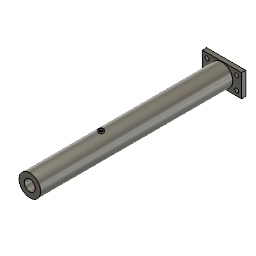
Full+System+Assembly (Autodesk Fusion 360 archive; units mm, degrees)
design "Measurement Tube"
Autodesk Fusion 360 part; units mm, degrees
note: some values were not read from the file. Set by a fixed rule: which face or edge a step refers to.
(part 1 of 5)
sketch "Sketch1" plane through (0, 0, 0) normal (0, 0, 1) x (1, 0, 0)
  circle A0 centre (0, 0) radius 6.375
  circle A1 centre (0, 0) radius 12.5
  dimension "d1" = 25
  dimension "d2" = 12.75
  constraint coincident A0.centre A1.centre
  measures "d1" diameter of A1
  measures "d2" diameter of A0
extrude "Extrude1" add sketch "Sketch1" along normal blind 225 contours A0 | A1
extrude "Extrude19" cut sketch "Sketch1" along normal up to surface (225 mm away) contours A0
sketch "Sketch22" plane through (0, 0, 0) normal (0, 0, 1) x (1, 0, 0)
  line L0 (22.5, 13) -> (-22.5, 13)
  line L1 (-22.5, 13) -> (-22.5, -13)
  line L2 (-22.5, -13) -> (22.5, -13)
  line L3 (22.5, -13) -> (22.5, 13)
  circle A0 centre (0, 0) radius 6.375 construction
  circle A1 centre (0, 0) radius 12.5 construction
  line L4 (0, 0) -> (22.5, 0) construction
  line L5 (0, 0) -> (-22.5, 0) construction
  circle A2 centre (0, 0) radius 12.5
  circle A3 centre (17, 7.5) radius 2.25
  circle A4 centre (-17, 7.5) radius 2.25
  circle A5 centre (-17, -7.5) radius 2.25
  circle A6 centre (17, -7.5) radius 2.25
  point P0 (12.5, 0)
  point P1 (-12.5, 0)
  dimension "d150" = 10
  dimension "d151" = 10
  dimension "d152" = 13
  dimension "d155" = 4.5
  dimension "d156" = 17
  dimension "d157" = 17
  dimension "d158" = 17
  dimension "d159" = 17
  dimension "d160" = 4.5
  dimension "d161" = 4.5
  dimension "d162" = 4.5
  dimension "d163" = 7.5
  dimension "d164" = 7.5
  dimension "d165" = 7.5
  dimension "d166" = 7.5
  constraint horizontal L0
  constraint vertical L1
  constraint horizontal L2
  constraint vertical L3
  constraint coincident A0.centre A1.centre
  constraint midpoint L3 L4.end
  constraint horizontal L4
  constraint coincident A1 P0
  constraint coincident L4 P0
  constraint midpoint L1 L5.end
  constraint coincident A1 P1
  constraint coincident L5 P1
  constraint coincident P0 A2
  measures "d150" distance of L4.end P0
  measures "d151" distance of L5.end P1
  measures "d152" distance of L0 A0.centre
  measures "d155" diameter of A3
  measures "d156" horizontal distance of A0.centre A3.centre
  measures "d157" horizontal distance of A0.centre A4.centre
  measures "d158" horizontal distance of A0.centre A6.centre
  measures "d159" horizontal distance of A0.centre A5.centre
  measures "d160" diameter of A4
  measures "d161" diameter of A6
  measures "d162" diameter of A5
  measures "d163" distance of L4 A3.centre
  measures "d164" distance of L5 A4.centre
  measures "d165" distance of L4 A6.centre
  measures "d166" distance of L5 A5.centre
extrude "Mount Holes" add sketch "Sketch22" along normal blind 5
ref_plane "WorkPlane4" through (0, 6.4, 0) normal (0, 1, 0) x (0, 0, 1)
sketch "Sketch21" plane through (0, 6.4, 0) normal (0, 1, 0) x (1, 0, 0)
  circle A0 centre (0, -143.363) radius 1.7
  circle A1 centre (0, -143.363) radius 2.7
  line L0 (-12.5, -225) -> (12.5, -225)
  line L1 (22.5, 0) -> (-22.5, 0) construction
  line L2 (-22.5, 0) -> (-22.5, -5) construction
  line L3 (-22.5, -5) -> (22.5, -5) construction
  line L4 (22.5, -5) -> (22.5, 0) construction
  line L5 (0, -5) -> (0, -225) construction
  dimension "d137" = 3.4
  dimension "d138" = 5.4
  dimension "d167" = 81.637
  constraint concentric A0 A1
  constraint midpoint L3 L5.start
  constraint midpoint L0 L5.end
  constraint coincident A0.centre L5
  measures "d137" diameter of A0
  measures "d138" diameter of A1
  measures "d167" distance of A0.centre L0
extrude "Extrude17" add sketch "Sketch21" along normal blind 8
extrude "Extrude18" cut sketch "Sketch21" along normal blind 8 and the other way blind 2 contours A0
equation "d5 = 12.8 mm"
equation "d20 = 0.105 in"
equation "d22 = d20"
equation "d29 = 2.5 in"
equation "d129 = 7.5 mm"
equation "d136 = d5 / 2"
equation "d138 = d137 + 2 mm"
equation "d151 = d150"
equation "d157 = d156"
equation "d158 = d156"
equation "d159 = d156"
equation "d160 = d155"
equation "d161 = d155"
equation "d162 = d155"
equation "d164 = d163"
equation "d165 = d163"
equation "d166 = d163"
equation "d50 = d48 / 2"
equation "d51 = d50"
equation "d52 = d53"
equation "d53 = d46 / 2"
equation "d54 = 4.25 mm"
equation "d55 = d54"
equation "d56 = -d45"
equation "d58 = 4.5 mm"
equation "d59 = d58"
equation "d64 = d67"
equation "d67 = 154.736 mm"
equation "d70 = d67"
equation "d110 = d26 / 2"
equation "d111 = d16 / 2"
equation "d115 = -d29"
equation "d119 = -d29"
equation "d127 = 17 mm"
equation "d128 = d127"
equation "d130 = d129"
equation "d131 = 4.25 mm"
equation "d132 = d131"

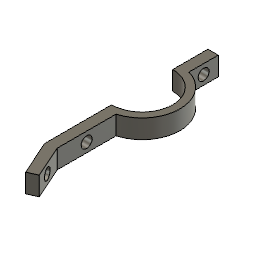
design "Trumpet Clamp 3 Secondary"
Autodesk Fusion 360 part; units mm, degrees
sketch "Sketch1" plane through (0, 0, 0) normal (0, 1, 0) x (1, 0, 0)
  circle A0 centre (0, 0) radius 12.435
  circle A1 centre (0, 0) radius 15.435
  line L0 (0, 0) -> (-15.435, 0) construction
  line L1 (0, 0) -> (15.435, 0) construction
  line L2 (-4.25, -40.647) -> (8.6182, -69.5153)
  line L3 (4.25, -38.8384) -> (16.3818, -66.0547)
  circle A2 centre (12.5, -67.785) radius 4.25
  line L4 (12.5, -67.785) -> (8.6182, -69.5153) construction
  line L5 (12.5, -67.785) -> (16.3818, -66.0547) construction
  circle A3 centre (12.5, -67.785) radius 2.25
  line L6 (-4.25, -40.647) -> (-4.25, -14.8384)
  line L7 (4.25, -38.8384) -> (4.25, -14.8384)
  line L8 (0, 0) -> (0, -38.8384) construction
  line L9 (4.25, -38.8384) -> (-4.25, -38.8384) construction
  line L10 (-4.25, 14.8384) -> (-4.25, 26.8384)
  line L11 (-4.25, 26.8384) -> (4.25, 26.8384)
  line L12 (4.25, 26.8384) -> (4.25, 14.8384)
  line L13 (-4.25, -14.8384) -> (-4.25, 14.8384) construction
  line L14 (4.25, 14.8384) -> (4.25, -14.8384) construction
  line L15 (12.5, -67.785) -> (12.5, -72.035) construction
  point P0 (0, -15.435)
  point P1 (12.5, -72.035)
  dimension "d1" = 24.87
  dimension "d3" = 4.5
  dimension "d4" = 8.5
  dimension "d5" = 12.5
  dimension "d19" = 8.5
  dimension "d22" = 30.87
  dimension "d31" = 12
  dimension "d32" = 24
  dimension "d35" = 56.6
  constraint coincident A0.centre A1.centre
  constraint concentric A0 A1
  constraint coincident A1 L0.end
  constraint horizontal L0
  constraint coincident A1 L1.end
  constraint parallel L0 L1
  constraint coincident A2.centre L4.start
  constraint coincident A2 L2.end
  constraint coincident A2 L3.end
  constraint parallel L4 L5
  constraint coincident L2.end L4.end
  constraint coincident L3.end L5.end
  constraint coincident A1 L6.end
  constraint coincident A1 L7.end
  constraint parallel L2 L3
  constraint vertical L6
  constraint vertical L7
  constraint vertical L8
  constraint tangent L3 A2
  constraint coincident L6 L9.end
  constraint perpendicular L6 L9
  constraint midpoint L8.end L9
  constraint coincident A1 L10.start
  constraint vertical L10
  constraint perpendicular L10 L11
  constraint coincident A1 L12.end
  constraint perpendicular L11 L12
  constraint vertical L13
  constraint vertical L14
  constraint coincident L8 P0
  constraint coincident A1 P0
  constraint coincident A2 P1
  constraint vertical L15
  constraint coincident P1 L15.end
  measures "d1" diameter of A0
  measures "d3" diameter of A3
  measures "d4" diameter of A2
  measures "d5" horizontal distance of A0.centre A2.centre
  measures "d19" distance of L6 L7
  measures "d22" diameter of A1
  measures "d31" distance of L11.end L12.end
  measures "d32" distance of L3.start L7.end
  measures "d35" vertical distance of P0 P1
extrude "Extrude1" add sketch "Sketch1" along normal blind 7.7
sketch "Sketch2" plane through (-10.8972, 0, 4.8575) normal (0.913367, 0, -0.407138) x (-0.407138, 0, -0.913367)
  line L0 (-67.0018, 0) -> (-37.204, 0)
  line L1 (-37.204, 0) -> (-37.204, 7.7)
  line L2 (-37.204, 7.7) -> (-67.0018, 7.7)
  line L3 (-67.0018, 7.7) -> (-67.0018, 0)
  line L4 (-37.204, 3.85) -> (-67.0018, 3.85) construction
  circle A0 centre (-45.204, 3.85) radius 2.25
  dimension "d33" = 8
  dimension "d34" = 4.5
  constraint midpoint L1 L4.start
  constraint midpoint L3 L4.end
  constraint coincident L4 A0.centre
  measures "d33" distance of L1 A0.centre
  measures "d34" diameter of A0
extrude "Extrude2" cut sketch "Sketch2" against normal up to surface (8.5 mm away) contours A0
sketch "Sketch3" plane through (4.25, 0, 0) normal (1, 0, 0) x (0, 0, -1)
  line L0 (-38.8384, 0) -> (-14.8384, 0)
  line L1 (-14.8384, 0) -> (-14.8384, 7.7)
  line L2 (-14.8384, 7.7) -> (-38.8384, 7.7)
  line L3 (-38.8384, 7.7) -> (-38.8384, 0)
  line L4 (-14.8384, 3.85) -> (-38.8384, 3.85) construction
  circle A0 centre (-26.8384, 3.85) radius 2.25
  line L5 (14.8384, 0) -> (26.8384, 0) construction
  line L6 (26.8384, 0) -> (26.8384, 7.7) construction
  line L7 (26.8384, 7.7) -> (14.8384, 7.7) construction
  line L8 (14.8384, 7.7) -> (14.8384, 0) construction
  line L9 (14.8384, 3.85) -> (26.8384, 3.85) construction
  circle A1 centre (20.8384, 3.85) radius 2.25
  dimension "d16" = 4.5
  constraint midpoint L1 L4.start
  constraint midpoint L3 L4.end
  constraint midpoint L4 A0.centre
  constraint midpoint L8 L9.start
  constraint midpoint L6 L9.end
  constraint midpoint L9 A1.centre
  constraint equal A0 A1
  measures "d16" diameter of A0
extrude "Extrude3" cut sketch "Sketch3" against normal up to surface (8.5 mm away) contours A0 | A1
sketch "Sketch4" plane through (0, 0, 0) normal (1, 0, 0) x (0, 0, -1)
  circle A0 centre (-26.8384, 3.85) radius 2.25 construction
  line L0 (-38.8384, 0) -> (-14.8384, 0) construction
  line L1 (-14.8384, 0) -> (-14.8384, 7.7) construction
  line L2 (-14.8384, 7.7) -> (-38.8384, 7.7) construction
  line L3 (-38.8384, 7.7) -> (-38.8384, 0) construction
  line L4 (14.8384, 0) -> (-14.8384, 0) construction
  line L5 (-14.8384, 0) -> (-14.8384, 7.7) construction
  line L6 (14.8384, 7.7) -> (-14.8384, 7.7) construction
  line L7 (-14.8384, 7.7) -> (-14.8384, 0) construction
  circle A1 centre (-26.8384, 3.85) radius 2.25 construction
  line L8 (-14.8384, 0) -> (-40.647, 0) construction
  line L9 (-40.647, 0) -> (-40.647, 7.7) construction
  line L10 (-40.647, 7.7) -> (-14.8384, 7.7) construction
  line L11 (-14.8384, 7.7) -> (-14.8384, 0) construction
  line L12 (14.8384, 0) -> (-39.7427, 0)
  line L13 (-39.7427, 0) -> (-39.7427, 7.7)
  line L14 (-39.7427, 7.7) -> (14.8384, 7.7)
  line L15 (14.8384, 7.7) -> (14.8384, 0)
  line L16 (-40.647, 7.7) -> (-38.8384, 7.7) construction
  line L17 (14.8384, 7.7) -> (14.8384, 0)
  line L18 (14.8384, 0) -> (-14.8384, 0)
  line L19 (14.8384, 0) -> (14.8384, 7.7)
  line L20 (14.8384, 7.7) -> (-14.8384, 7.7)
  circle A2 centre (20.8384, 3.85) radius 2.25
  line L21 (14.8384, 0) -> (26.8384, 0)
  line L22 (26.8384, 0) -> (26.8384, 7.7)
  line L23 (26.8384, 7.7) -> (14.8384, 7.7)
  line L24 (14.8384, 7.7) -> (14.8384, 0)
  constraint horizontal L12
  constraint vertical L13
  constraint horizontal L14
  constraint vertical L15
  constraint coincident L10 L13.end
  constraint coincident L4.start L12.start
  constraint coincident L9.end L10.start
  constraint coincident L2.end L3.start
  constraint midpoint L13.end L16
extrude "Extrude4" cut sketch "Sketch4" against normal blind 15.435
ref_plane "WorkPlane1" through (6.0659, 3.85, 53.3509) normal (-0.913367, 0, 0.407138) x (0.407138, 0, 0.913367)
sketch "Sketch5" plane through (-14.779, 0, 6.5878) normal (-0.913367, 0, 0.407138) x (0.407138, 0, 0.913367)
  line L0 (11.3577, 7.7) -> (11.3577, 0) construction
  line L1 (11.3577, 0) -> (36.2997, 0) construction
  line L2 (36.2997, 0) -> (36.2997, 7.7) construction
  line L3 (36.2997, 7.7) -> (11.3577, 7.7) construction
  ellipse E0 centre (24.5133, 3.85) end of major axis (24.5133, 1.6) minor radius 2.0551
  line L4 (64.7518, 7.7) -> (69.2518, 7.7) construction
  line L5 (36.2997, 7.7) -> (67.0018, 7.7) construction
  line L6 (67.0018, 7.7) -> (67.0018, 0) construction
  line L7 (67.0018, 0) -> (36.2997, 0) construction
  line L8 (36.2997, 0) -> (36.2997, 7.7) construction
  line L9 (51.6507, 7.7) -> (33.5308, 7.7)
  line L10 (33.5308, 7.7) -> (33.5308, 0)
  line L11 (33.5308, 0) -> (51.6507, 0)
  line L12 (51.6507, 0) -> (51.6507, 7.7)
  constraint horizontal L5
  constraint vertical L6
  constraint horizontal L7
  constraint vertical L8
  constraint coincident L2.end L3.start
  constraint midpoint L4 L5.end
  constraint coincident L1.end L7
  constraint horizontal L9
  constraint vertical L10
  constraint horizontal L11
  constraint vertical L12
  constraint coincident L1 L10.end
  constraint midpoint L5 L9.start
extrude "Extrude5" cut sketch "Sketch5" along normal up to surface (4.25 mm away) contours L9 L10 L11 L12
sketch "Sketch6" plane through (-18.6608, 0, 8.3181) normal (-0.913367, 0, 0.407138) x (0.407138, 0, 0.913367)
  line L0 (36.2997, 7.7) -> (36.2997, 0)
  line L1 (36.2997, 0) -> (51.6507, 0)
  line L2 (51.6507, 7.7) -> (36.2997, 7.7)
  circle A0 centre (45.204, 3.85) radius 2.25
  line L3 (51.6507, 7.7) -> (111.7151, 7.7)
  line L4 (111.7151, 7.7) -> (111.7151, 0)
  line L5 (111.7151, 0) -> (51.6507, 0)
  line L6 (51.6507, 0) -> (51.6507, 7.7)
  line L7 (51.6507, 0) -> (51.6507, 7.7)
  constraint horizontal L3
  constraint vertical L4
  constraint horizontal L5
  constraint vertical L6
  constraint coincident L2.start L3.start
  constraint coincident L1.end L5
extrude "Extrude6" cut sketch "Sketch6" against normal up to surface (8.5 mm away) contours L3 L4 L5 L6 L7
equation "d19 = d4"
equation "d20 = ( -d22 / 2 mm ) * 1 mm"
equation "d22 = d1 + 6 mm"

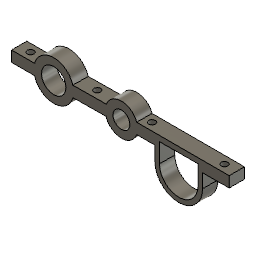
design "Trumpet Mount Close"
Autodesk Fusion 360 part; units mm, degrees
sketch "Sketch1" plane through (0, 0, 0) normal (0, 0, 1) x (1, 0, 0)
  circle A0 centre (-43.925, 0) radius 12.925
  circle A1 centre (-43.925, 0) radius 7.925
  circle A2 centre (0, 0) radius 10.5
  circle A3 centre (0, 0) radius 5.5
  line L0 (9.8995, 3.5) -> (69.8995, 3.5)
  line L1 (69.8995, 3.5) -> (69.8995, -3.5)
  line L2 (69.8995, -3.5) -> (9.8995, -3.5)
  line L3 (-31.5162, 3.6163) -> (-9.7806, 3.8197)
  line L4 (-31.4507, -3.3834) -> (-10.006, -3.1827)
  line L5 (-56.3671, 3.5) -> (-71.3671, 3.5)
  line L6 (-71.3671, 3.5) -> (-71.3671, -3.5)
  line L7 (-71.3671, -3.5) -> (-56.3671, -3.5)
  line L8 (-43.925, 0) -> (0, 0) construction
  dimension "d1" = 3.5
  dimension "d2" = 3.5
  dimension "d3" = 3.5
  dimension "d4" = 3.5
  dimension "d5" = 3.5
  dimension "d6" = 3.5
  dimension "d7" = 43.925
  dimension "d8" = 60
  dimension "d9" = 15
  dimension "d19" = 25.85
  dimension "d20" = 21
  dimension "d21" = 11
  dimension "d22" = 15.85
  constraint concentric A0 A1
  constraint concentric A2 A3
  constraint coincident A2 L0.start
  constraint horizontal L0
  constraint perpendicular L0 L1
  constraint coincident A2 L2.end
  constraint perpendicular L1 L2
  constraint coincident A0 L3.start
  constraint coincident A2 L3.end
  constraint coincident A0 L4.start
  constraint coincident A2 L4.end
  constraint parallel L3 L4
  constraint coincident A0 L5.start
  constraint horizontal L5
  constraint perpendicular L5 L6
  constraint coincident A0 L7.end
  constraint perpendicular L6 L7
  constraint coincident A0.centre A1.centre
  constraint coincident A2.centre A3.centre
  constraint horizontal L8
  measures "d1" distance of A2.centre L2
  measures "d2" distance of A2.centre L0
  measures "d3" distance of A0.centre L3
  measures "d4" distance of A0.centre L4
  measures "d5" distance of A0.centre L7
  measures "d6" distance of A0.centre L5
  measures "d7" horizontal distance of A0.centre A2.centre
  measures "d8" distance of L0.start L0.end
  measures "d9" distance of L5.start L5.end
  measures "d19" diameter of A0
  measures "d20" diameter of A2
  measures "d21" diameter of A3
  measures "d22" diameter of A1
extrude "Extrude1" add sketch "Sketch1" along normal mid plane 10
sketch "Sketch4" plane through (0, 3.5, 0) normal (0, 1, 0) x (-1, 0, 0)
  line L0 (71.3671, -5) -> (71.3671, 5)
  line L1 (71.3671, 5) -> (56.3671, 5)
  line L2 (56.3671, 5) -> (56.3671, -5)
  line L3 (56.3671, -5) -> (71.3671, -5)
  circle A0 centre (63.8671, 0) radius 2.125
  line L4 (31.5162, -5) -> (9.7806, -5)
  line L5 (31.5162, 5) -> (31.5162, -5)
  line L6 (9.7806, -5) -> (9.7806, 5)
  dimension "d25" = 4.25
  dimension "d27" = 5
  dimension "d31" = 7.5
  dimension "d32" = 7.5
  measures "d25" diameter of A0
  measures "d27" distance of L3 A0.centre
  measures "d31" distance of L0 A0.centre
  measures "d32" distance of L2 A0.centre
extrude "Extrude4" cut sketch "Sketch4" along normal up to surface contours A0 end surface through (-31.4507, -3.3834, 0) normal (0.009359, -0.999956, 0) offset 0
sketch "Sketch5" plane through (-0.0366, 3.9109, 0) normal (-0.009359, 0.999956, 0) x (0, 0, 1)
  line L0 (-5, -31.481) -> (5, -31.481)
  line L1 (5, -31.481) -> (5, -9.7444)
  line L2 (5, -9.7444) -> (-5, -9.7444)
  line L3 (-5, -9.7444) -> (-5, -31.481)
  circle A0 centre (0, -20.613) radius 2.125
  dimension "d35" = 4.25
  dimension "d36" = 10.868
  dimension "d37" = 10.8686
  dimension "d38" = 5
  measures "d35" diameter of A0
  measures "d36" distance of L0 A0.centre
  measures "d37" distance of L2 A0.centre
  measures "d38" distance of L3 A0.centre
extrude "Extrude5" cut sketch "Sketch5" against normal up to surface (7 mm away) contours A0
sketch "Sketch6" plane through (0, 3.5, 0) normal (0, 1, 0) x (-1, 0, 0)
  line L0 (-9.8995, -5) -> (-9.8995, 5)
  line L1 (-9.8995, 5) -> (-69.8995, 5)
  line L2 (-69.8995, 5) -> (-69.8995, -5)
  line L3 (-69.8995, -5) -> (-9.8995, -5)
sketch "Sketch7" plane through (0, 3.5, 0) normal (0, 1, 0) x (-1, 0, 0)
  line L0 (-9.8995, -5) -> (-9.8995, 5) construction
  line L1 (-9.8995, 5) -> (-69.8995, 5) construction
  line L2 (-69.8995, 5) -> (-69.8995, -5) construction
  line L3 (-69.8995, -5) -> (-9.8995, -5) construction
  line L4 (-69.8995, 0) -> (-9.8995, 0) construction
  circle A0 centre (-61.8995, 0) radius 2.125
  circle A1 centre (-14.8995, 0) radius 2.125
  dimension "d41" = 4.25
  dimension "d42" = 4.25
  dimension "d43" = 8
  dimension "d44" = 5
  constraint midpoint L2 L4.start
  constraint midpoint L0 L4.end
  constraint coincident L4 A0.centre
  constraint coincident L4 A1.centre
  measures "d41" diameter of A0
  measures "d42" diameter of A1
  measures "d43" distance of L2 A0.centre
  measures "d44" distance of L0 A1.centre
extrude "Extrude6" cut sketch "Sketch7" against normal up to surface (7 mm away)
sketch "Sketch8" plane through (0, 0, 5) normal (0, 0, 1) x (1, 0, 0)
  line L0 (-71.3671, 3.5) -> (-71.3671, -3.5)
  line L1 (-71.3671, -3.5) -> (-56.3671, -3.5)
  arc A0 (-56.3671, -3.5) -> (-31.4507, -3.3834) centre (-43.925, 0) ccw
  line L2 (-31.4507, -3.3834) -> (-10.006, -3.1827)
  arc A1 (-10.006, -3.1827) -> (9.8995, -3.5) centre (0, 0) ccw
  line L3 (9.8995, -3.5) -> (69.8995, -3.5)
  line L4 (69.8995, -3.5) -> (69.8995, 3.5)
  line L5 (52.6495, 0) -> (52.6495, -28) construction
  line L6 (52.6495, -28) -> (21.6495, -28) construction
  line L7 (21.6495, -28) -> (21.6495, 0) construction
  circle A2 centre (37.1495, -12.5) radius 12.5 construction
  line L8 (37.1495, -12.5) -> (37.1495, 0) construction
  line L9 (37.1495, -12.5) -> (52.6495, -12.5) construction
  line L10 (37.1495, -12.5) -> (21.6495, -12.5) construction
  line L11 (24.6495, -12.5) -> (24.6495, 0)
  line L12 (49.6495, -12.5) -> (49.6495, 0)
  arc A3 (24.6495, -12.5) -> (49.6495, -12.5) centre (37.1495, -12.5) ccw
  arc A4 (21.6495, -12.5) -> (37.1495, -28) centre (37.1495, -12.5) ccw
  arc A5 (37.1495, -28) -> (52.6495, -12.5) centre (37.1495, -12.5) ccw
  line L13 (21.6495, -12.5) -> (21.6495, 0)
  line L14 (52.6495, -12.5) -> (52.6495, 0)
  line L15 (21.6495, 0) -> (52.6495, 0)
  circle A6 centre (-43.925, 0) radius 7.925
  circle A7 centre (0, 0) radius 5.5
  arc A8 (-31.5162, 3.6163) -> (-56.3671, 3.5) centre (-43.925, 0) ccw
  line L16 (-56.3671, 3.5) -> (-71.3671, 3.5)
  line L17 (69.8995, 3.5) -> (9.8995, 3.5)
  arc A9 (9.8995, 3.5) -> (-9.7806, 3.8197) centre (0, 0) ccw
  line L18 (-9.7806, 3.8197) -> (-31.5162, 3.6163)
  point P0 (37.1495, 0)
  dimension "d49" = 17.25
  dimension "d50" = 31
  dimension "d51" = 28
  dimension "d52" = 25
  constraint vertical L5
  constraint horizontal L6
  constraint vertical L7
  constraint coincident A2.centre L8.start
  constraint coincident L8 P0
  constraint coincident A2 P0
  constraint coincident L5 L9.end
  constraint perpendicular L5 L9
  constraint coincident L7 L10.end
  constraint perpendicular L7 L10
  constraint coincident A2 L11.start
  constraint coincident L10 L11.start
  constraint tangent A2 L11
  constraint coincident A2 L12.start
  constraint coincident L9 L12.start
  constraint tangent A2 L12
  constraint tangent L12 A3
  constraint tangent L6 A4
  constraint coincident L6 A4.end
  constraint tangent L5 A5
  constraint perpendicular L14 L15
  constraint coincident L11.end L15
  constraint coincident L12.end L15
  constraint coincident P0 L15
  constraint midpoint P0 L15
  measures "d49" distance of L4 L5
  measures "d50" distance of L7.end L5.start
  measures "d51" distance of L5.start L5.end
  measures "d52" diameter of A2
extrude "Extrude7" add sketch "Sketch8" against normal up to surface (10 mm away) contours L3 L11 L12 A3 A4 A5 L13 L14
sketch "Sketch9" plane through (0, 0, 5) normal (0, 0, 1) x (1, 0, 0)
  line L0 (24.6495, -3.5) -> (49.6495, -3.5)
  line L1 (49.6495, -3.5) -> (49.6495, -12.5)
  arc A0 (24.6495, -12.5) -> (49.6495, -12.5) centre (37.1495, -12.5) ccw
  line L2 (24.6495, -12.5) -> (24.6495, -3.5)
  line L3 (21.6495, -3.5) -> (21.6495, -12.5)
  arc A1 (21.6495, -12.5) -> (37.1495, -28) centre (37.1495, -12.5) ccw
  line L4 (52.6495, -12.5) -> (52.6495, -3.5)
  line L5 (52.6495, -3.5) -> (69.8995, -3.5)
  line L6 (69.8995, -3.5) -> (69.8995, 3.5)
  line L7 (-71.3671, 3.5) -> (-71.3671, -3.5)
  line L8 (-71.3671, -3.5) -> (-56.3671, -3.5)
  arc A2 (-56.3671, -3.5) -> (-31.4507, -3.3834) centre (-43.925, 0) ccw
  line L9 (-31.4507, -3.3834) -> (-10.006, -3.1827)
  arc A3 (-10.006, -3.1827) -> (9.8995, -3.5) centre (0, 0) ccw
  line L10 (9.8995, -3.5) -> (21.6495, -3.5)
  line L11 (24.6495, -3.5) -> (49.6495, -3.5)
  line L12 (49.6495, -3.5) -> (49.6495, 0)
  line L13 (49.6495, 0) -> (24.6495, 0)
  line L14 (24.6495, 0) -> (24.6495, -3.5)
  line L15 (49.6495, -6.9259) -> (49.6495, 0) construction
  arc A4 (37.1495, -28) -> (52.6495, -12.5) centre (37.1495, -12.5) ccw
  circle A5 centre (-43.925, 0) radius 7.925
  circle A6 centre (0, 0) radius 5.5
  line L16 (69.8995, 3.5) -> (9.8995, 3.5)
  arc A7 (9.8995, 3.5) -> (-9.7806, 3.8197) centre (0, 0) ccw
  line L17 (-9.7806, 3.8197) -> (-31.5162, 3.6163)
  arc A8 (-31.5162, 3.6163) -> (-56.3671, 3.5) centre (-43.925, 0) ccw
  line L18 (-56.3671, 3.5) -> (-71.3671, 3.5)
  constraint horizontal L11
  constraint vertical L12
  constraint horizontal L13
  constraint vertical L14
  constraint coincident L0.start L2.end
  constraint coincident L1 L15.start
  constraint perpendicular L13 L15
extrude "Extrude8" cut sketch "Sketch9" against normal up to surface (10 mm away) contours L0 L11 L12 L13 L14
sketch "Sketch3" plane through (0, 0, 0) normal (0, 1, 0) x (1, 0, 0)
  line L0 (-71.3671, 5) -> (-71.3671, -5)
  line L1 (-71.3671, -5) -> (-56.3671, -5)
  line L2 (-56.3671, -5) -> (-56.3671, 5)
  line L3 (-56.3671, 5) -> (-71.3671, 5)
  line L4 (9.8995, 5) -> (9.8995, -5)
  line L5 (9.8995, -5) -> (69.8995, -5)
  line L6 (69.8995, -5) -> (69.8995, 5)
  line L7 (69.8995, 5) -> (9.8995, 5)
  line L8 (-71.3671, 5) -> (69.8995, 5)
  line L9 (69.8995, 5) -> (69.8995, -5)
  line L10 (69.8995, -5) -> (-71.3671, -5)
  line L11 (-71.3671, -5) -> (-71.3671, 5)
  circle A0 centre (-63.8671, 0) radius 2.125
  circle A1 centre (14.8995, 0) radius 2.125
  circle A2 centre (61.8995, 0) radius 2.125
  constraint horizontal L8
  constraint vertical L9
  constraint horizontal L10
  constraint vertical L11
  constraint coincident L5.end L6.start
  constraint coincident L0.start L3.end
extrude "Extrude3" [rolled back] along distance 20 taper angle 0
equation "d2 = d1"
equation "d3 = d1"
equation "d4 = d1"
equation "d5 = d1"
equation "d6 = d1"
equation "d42 = d41"
equation "d49 = 20.25 mm - 3 mm"
equation "d50 = 25 mm + 6 mm"
equation "d51 = 25 mm + 3 mm"

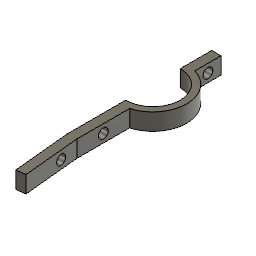
design "Trumpet Clamp 2 Secondary"
Autodesk Fusion 360 part; units mm, degrees
sketch "Sketch1" plane through (0, 0, 0) normal (0, 1, 0) x (1, 0, 0)
  circle A0 centre (0, 0) radius 12.435
  circle A1 centre (0, 0) radius 15.435
  line L0 (0, 0) -> (-15.435, 0) construction
  line L1 (0, 0) -> (15.435, 0) construction
  line L2 (-4.25, -39.2475) -> (0.7697, -91.2632)
  line L3 (4.25, -38.8384) -> (9.2303, -90.4468)
  circle A2 centre (5, -90.855) radius 4.25
  line L4 (5, -90.855) -> (0.7697, -91.2632) construction
  line L5 (5, -90.855) -> (9.2303, -90.4468) construction
  circle A3 centre (5, -90.855) radius 2.25
  line L6 (-4.25, -39.2475) -> (-4.25, -14.8384)
  line L7 (4.25, -38.8384) -> (4.25, -14.8384)
  line L8 (0, 0) -> (0, -38.8384) construction
  line L9 (4.25, -38.8384) -> (-4.25, -38.8384) construction
  line L10 (-4.25, 14.8384) -> (-4.25, 26.8384)
  line L11 (-4.25, 26.8384) -> (4.25, 26.8384)
  line L12 (4.25, 26.8384) -> (4.25, 14.8384)
  line L13 (-4.25, -14.8384) -> (-4.25, 14.8384) construction
  line L14 (4.25, 14.8384) -> (4.25, -14.8384) construction
  line L15 (5, -90.855) -> (5, -95.105) construction
  point P0 (0, -15.435)
  point P1 (5, -95.105)
  dimension "d1" = 24.87
  dimension "d3" = 4.5
  dimension "d4" = 8.5
  dimension "d5" = 5
  dimension "d19" = 8.5
  dimension "d22" = 30.87
  dimension "d31" = 12
  dimension "d32" = 24
  dimension "d35" = 79.67
  constraint coincident A0.centre A1.centre
  constraint concentric A0 A1
  constraint coincident A1 L0.end
  constraint horizontal L0
  constraint coincident A1 L1.end
  constraint parallel L0 L1
  constraint coincident A2.centre L4.start
  constraint coincident A2 L2.end
  constraint coincident A2 L3.end
  constraint parallel L4 L5
  constraint coincident L2.end L4.end
  constraint coincident L3.end L5.end
  constraint coincident A1 L6.end
  constraint coincident A1 L7.end
  constraint parallel L2 L3
  constraint vertical L6
  constraint vertical L7
  constraint vertical L8
  constraint tangent L3 A2
  constraint coincident L6 L9.end
  constraint perpendicular L6 L9
  constraint midpoint L8.end L9
  constraint coincident A1 L10.start
  constraint vertical L10
  constraint perpendicular L10 L11
  constraint coincident A1 L12.end
  constraint perpendicular L11 L12
  constraint vertical L13
  constraint vertical L14
  constraint coincident L8 P0
  constraint coincident A1 P0
  constraint coincident A2 P1
  constraint vertical L15
  constraint coincident P1 L15.end
  measures "d1" diameter of A0
  measures "d3" diameter of A3
  measures "d4" diameter of A2
  measures "d5" horizontal distance of A0.centre A2.centre
  measures "d19" distance of L6 L7
  measures "d22" diameter of A1
  measures "d31" distance of L11.end L12.end
  measures "d32" distance of L3.start L7.end
  measures "d35" vertical distance of P0 P1
extrude "Extrude1" add sketch "Sketch1" along normal blind 7.7
sketch "Sketch2" plane through (0.4974, 0, -0.048) normal (0.995376, 0, -0.096056) x (-0.096056, 0, -0.995376)
  line L0 (-90.9152, 0) -> (-39.067, 0)
  line L1 (-39.067, 0) -> (-39.067, 7.7)
  line L2 (-39.067, 7.7) -> (-90.9152, 7.7)
  line L3 (-90.9152, 7.7) -> (-90.9152, 0)
  line L4 (-39.067, 3.85) -> (-90.9152, 3.85) construction
  circle A0 centre (-47.067, 3.85) radius 2.25
  dimension "d33" = 8
  dimension "d34" = 4.5
  constraint midpoint L1 L4.start
  constraint midpoint L3 L4.end
  constraint coincident L4 A0.centre
  measures "d33" distance of L1 A0.centre
  measures "d34" diameter of A0
extrude "Extrude2" cut sketch "Sketch2" against normal up to surface (8.5 mm away) contours A0
sketch "Sketch3" plane through (4.25, 0, 0) normal (1, 0, 0) x (0, 0, -1)
  line L0 (-38.8384, 0) -> (-14.8384, 0)
  line L1 (-14.8384, 0) -> (-14.8384, 7.7)
  line L2 (-14.8384, 7.7) -> (-38.8384, 7.7)
  line L3 (-38.8384, 7.7) -> (-38.8384, 0)
  line L4 (-14.8384, 3.85) -> (-38.8384, 3.85) construction
  circle A0 centre (-26.8384, 3.85) radius 2.25
  line L5 (14.8384, 0) -> (26.8384, 0) construction
  line L6 (26.8384, 0) -> (26.8384, 7.7) construction
  line L7 (26.8384, 7.7) -> (14.8384, 7.7) construction
  line L8 (14.8384, 7.7) -> (14.8384, 0) construction
  line L9 (14.8384, 3.85) -> (26.8384, 3.85) construction
  circle A1 centre (20.8384, 3.85) radius 2.25
  dimension "d16" = 4.5
  constraint midpoint L1 L4.start
  constraint midpoint L3 L4.end
  constraint midpoint L4 A0.centre
  constraint midpoint L8 L9.start
  constraint midpoint L6 L9.end
  constraint midpoint L9 A1.centre
  constraint equal A0 A1
  measures "d16" diameter of A0
extrude "Extrude3" cut sketch "Sketch3" against normal up to surface (8.5 mm away) contours A0 | A1
sketch "Sketch4" plane through (0, 0, 0) normal (1, 0, 0) x (0, 0, -1)
  circle A0 centre (-26.8384, 3.85) radius 2.25 construction
  line L0 (-38.8384, 0) -> (-14.8384, 0) construction
  line L1 (-14.8384, 0) -> (-14.8384, 7.7) construction
  line L2 (-14.8384, 7.7) -> (-38.8384, 7.7) construction
  line L3 (-38.8384, 7.7) -> (-38.8384, 0) construction
  line L4 (14.8384, 0) -> (-14.8384, 0) construction
  line L5 (-14.8384, 0) -> (-14.8384, 7.7) construction
  line L6 (14.8384, 7.7) -> (-14.8384, 7.7) construction
  line L7 (-14.8384, 7.7) -> (-14.8384, 0) construction
  circle A1 centre (-26.8384, 3.85) radius 2.25 construction
  line L8 (-14.8384, 0) -> (-39.2475, 0) construction
  line L9 (-39.2475, 0) -> (-39.2475, 7.7) construction
  line L10 (-39.2475, 7.7) -> (-14.8384, 7.7) construction
  line L11 (-14.8384, 7.7) -> (-14.8384, 0) construction
  line L12 (14.8384, 0) -> (-39.0429, 0)
  line L13 (-39.0429, 0) -> (-39.0429, 7.7)
  line L14 (-39.0429, 7.7) -> (14.8384, 7.7)
  line L15 (14.8384, 7.7) -> (14.8384, 0)
  line L16 (-39.2475, 7.7) -> (-38.8384, 7.7) construction
  line L17 (14.8384, 7.7) -> (14.8384, 0)
  line L18 (14.8384, 0) -> (-14.8384, 0)
  line L19 (14.8384, 0) -> (14.8384, 7.7)
  line L20 (14.8384, 7.7) -> (-14.8384, 7.7)
  circle A2 centre (20.8384, 3.85) radius 2.25
  line L21 (14.8384, 0) -> (26.8384, 0)
  line L22 (26.8384, 0) -> (26.8384, 7.7)
  line L23 (26.8384, 7.7) -> (14.8384, 7.7)
  line L24 (14.8384, 7.7) -> (14.8384, 0)
  constraint horizontal L12
  constraint vertical L13
  constraint horizontal L14
  constraint vertical L15
  constraint coincident L10 L13.end
  constraint coincident L4.start L12.start
  constraint coincident L9.end L10.start
  constraint coincident L2.end L3.start
  constraint midpoint L13.end L16
extrude "Extrude4" cut sketch "Sketch4" against normal blind 15.435
ref_plane "WorkPlane1" through (2.4902, 3.85, 64.8471) normal (-0.995376, 0, 0.096056) x (0.096056, 0, 0.995376)
sketch "Sketch5" plane through (-3.733, 0, 0.3602) normal (-0.995376, 0, 0.096056) x (0.096056, 0, 0.995376)
  line L0 (12.3775, 7.7) -> (12.3775, 0) construction
  line L1 (12.3775, 0) -> (38.8624, 0) construction
  line L2 (38.8624, 0) -> (38.8624, 7.7) construction
  line L3 (38.8624, 7.7) -> (12.3775, 7.7) construction
  ellipse E0 centre (26.7142, 3.85) end of major axis (26.7142, 1.6) minor radius 2.2396
  line L4 (88.6652, 7.7) -> (93.1652, 7.7) construction
  line L5 (38.8624, 7.7) -> (90.9152, 7.7) construction
  line L6 (90.9152, 7.7) -> (90.9152, 0) construction
  line L7 (90.9152, 0) -> (38.8624, 0) construction
  line L8 (38.8624, 0) -> (38.8624, 7.7) construction
  line L9 (64.8888, 7.7) -> (33.5308, 7.7)
  line L10 (33.5308, 7.7) -> (33.5308, 0)
  line L11 (33.5308, 0) -> (64.8888, 0)
  line L12 (64.8888, 0) -> (64.8888, 7.7)
  constraint horizontal L5
  constraint vertical L6
  constraint horizontal L7
  constraint vertical L8
  constraint coincident L2.end L3.start
  constraint midpoint L4 L5.end
  constraint coincident L1.end L7
  constraint horizontal L9
  constraint vertical L10
  constraint horizontal L11
  constraint vertical L12
  constraint coincident L1 L10.end
  constraint midpoint L5 L9.start
extrude "Extrude5" cut sketch "Sketch5" along normal up to surface (4.25 mm away) contours L9 L10 L11 L12
sketch "Sketch6" plane through (-7.9633, 0, 0.7685) normal (-0.995376, 0, 0.096056) x (0.096056, 0, 0.995376)
  line L0 (38.8624, 7.7) -> (38.8624, 0)
  line L1 (38.8624, 0) -> (64.8888, 0)
  line L2 (64.8888, 7.7) -> (38.8624, 7.7)
  circle A0 centre (47.067, 3.85) radius 2.25
  line L3 (64.8888, 7.7) -> (111.7152, 7.7)
  line L4 (111.7152, 7.7) -> (111.7152, 0)
  line L5 (111.7152, 0) -> (64.8888, 0)
  line L6 (64.8888, 0) -> (64.8888, 7.7)
  line L7 (64.8888, 0) -> (64.8888, 7.7)
  constraint horizontal L3
  constraint vertical L4
  constraint horizontal L5
  constraint vertical L6
  constraint coincident L2.start L3.start
  constraint coincident L1.end L5
extrude "Extrude6" cut sketch "Sketch6" against normal up to surface (8.5 mm away) contours L3 L4 L5 L6 L7
equation "d19 = d4"
equation "d20 = ( -d22 / 2 mm ) * 1 mm"
equation "d22 = d1 + 6 mm"

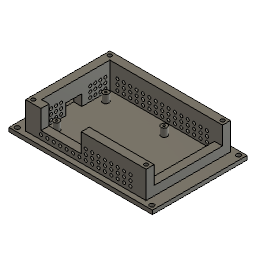
design "RPi Board Case"
Autodesk Fusion 360 part; units mm, degrees
sketch "Sketch1" plane through (0, 0, 0) normal (0, 1, 0) x (1, 0, 0)
  line L0 (-60, 42) -> (60, 42)
  line L1 (60, 42) -> (60, -42)
  line L2 (60, -42) -> (-60, -42)
  line L3 (-60, -42) -> (-60, 42)
  dimension "d1" = 120
  dimension "d2" = 84
  dimension "d3" = 60
  dimension "d4" = 42
  constraint horizontal L0
  constraint vertical L1
  constraint horizontal L2
  constraint vertical L3
  measures "d1" distance of L0.start L0.end
  measures "d2" distance of L0.start L2.end
  measures "d3" distance of origin L1
  measures "d4" distance of origin L0
extrude "Extrude1" add sketch "Sketch1" along normal blind 5 makes body 1
sketch "Sketch2" plane through (0, 5, 0) normal (0, 1, 0) x (-1, 0, 0)
  line L0 (60, 42) -> (-60, 42)
  line L1 (-60, 42) -> (-60, -42)
  line L2 (-60, -42) -> (60, -42)
  line L3 (60, -42) -> (60, 42)
  line L4 (52, -34) -> (-52, -34)
  line L5 (-52, -34) -> (-52, 34)
  line L6 (-52, 34) -> (52, 34)
  line L7 (52, 34) -> (52, -34)
  dimension "d7" = 8
  dimension "d8" = 8
  dimension "d9" = 8
  dimension "d10" = 8
  constraint horizontal L4
  constraint vertical L5
  constraint horizontal L6
  constraint vertical L7
  measures "d7" distance of L3 L7
  measures "d8" distance of L2 L4
  measures "d9" distance of L1 L5
  measures "d10" distance of L0 L6
extrude "Extrude2" add sketch "Sketch2" along normal blind 26 bodies 1
sketch "Sketch3" plane through (0, 5, 0) normal (0, 1, 0) x (-1, 0, 0)
  line L0 (-52, 34) -> (-52, -34)
  line L1 (-52, -34) -> (52, -34)
  line L2 (52, -34) -> (52, 34)
  line L3 (52, 34) -> (-52, 34)
  line L4 (44.5, -22.5) -> (-13.5, -22.5) construction
  line L5 (-13.5, -22.5) -> (-13.5, 26.5) construction
  line L6 (-13.5, 26.5) -> (44.5, 26.5) construction
  line L7 (44.5, 26.5) -> (44.5, -22.5) construction
  circle A0 centre (44.5, -22.5) radius 1.05
  circle A1 centre (-13.5, -22.5) radius 1.05
  circle A2 centre (-13.5, 26.5) radius 1.05
  circle A3 centre (44.5, 26.5) radius 1.05
  circle A4 centre (44.5, -22.5) radius 3.05
  circle A5 centre (-13.5, -22.5) radius 3.05
  circle A6 centre (-13.5, 26.5) radius 3.05
  circle A7 centre (44.5, 26.5) radius 3.05
  dimension "d13" = 58
  dimension "d14" = 49
  dimension "d15" = 11.5
  dimension "d16" = 7.5
  dimension "d17" = 2.1
  dimension "d18" = 2.1
  dimension "d19" = 2.1
  dimension "d20" = 2.1
  dimension "d21" = 6.1
  dimension "d22" = 6.1
  dimension "d23" = 6.1
  dimension "d24" = 6.1
  dimension "d50" = 38.5
  constraint horizontal L4
  constraint vertical L5
  constraint horizontal L6
  constraint vertical L7
  constraint coincident L4.start L7.end
  constraint coincident L4.end L5.start
  constraint coincident L5.end L6.start
  constraint coincident L6.end L7.start
  constraint concentric A0 A4
  constraint concentric A1 A5
  constraint concentric A2 A6
  constraint concentric A3 A7
  measures "d13" distance of L4.start L4.end
  measures "d14" distance of L4.start L6.end
  measures "d15" distance of L1 L4
  measures "d16" distance of L2 L7
  measures "d17" diameter of A0
  measures "d18" diameter of A1
  measures "d19" diameter of A2
  measures "d20" diameter of A3
  measures "d21" diameter of A4
  measures "d22" diameter of A5
  measures "d23" diameter of A6
  measures "d24" diameter of A7
  measures "d50" distance of L0 L5
extrude "Extrude3" add sketch "Sketch3" along normal blind 8 contours A4 | A5 | A6 | A7 bodies 1
sketch "Sketch4" plane through (0, 0, 42) normal (0, 0, 1) x (1, 0, 0)
  line L0 (-60, 0) -> (60, 0)
  line L1 (60, 0) -> (60, 31)
  line L2 (60, 31) -> (-60, 31)
  line L3 (-60, 31) -> (-60, 0)
  line L4 (-47.55, 5) -> (-41.45, 5)
  line L5 (10.45, 5) -> (16.55, 5)
  line L6 (52, 5) -> (-52, 5)
  line L7 (-52, 5) -> (52, 5)
  line L8 (10.45, 5) -> (16.55, 5)
  line L9 (-47.55, 5) -> (-41.45, 5)
  line L10 (-44.5, 32) -> (-4.5, 32)
  line L11 (-4.5, 32) -> (-4.5, 12)
  line L12 (-4.5, 12) -> (-44.5, 12)
  line L13 (-44.5, 12) -> (-44.5, 32)
  line L14 (-44.5, 12) -> (-44.5, 5) construction
  circle A0 centre (-44.5, 8.5) radius 1.5
  circle A1 centre (-38.1429, 8.5) radius 1.5
  circle A2 centre (-31.7857, 8.5) radius 1.5
  circle A3 centre (-25.4286, 8.5) radius 1.5
  circle A4 centre (-19.0714, 8.5) radius 1.5
  circle A5 centre (-12.7143, 8.5) radius 1.5
  circle A6 centre (-6.3571, 8.5) radius 1.5
  circle A7 centre (0, 8.5) radius 1.5
  circle A8 centre (6.3571, 8.5) radius 1.5
  circle A9 centre (12.7143, 8.5) radius 1.5
  circle A10 centre (19.0714, 8.5) radius 1.5
  circle A11 centre (25.4286, 8.5) radius 1.5
  circle A12 centre (31.7857, 8.5) radius 1.5
  circle A13 centre (38.1429, 8.5) radius 1.5
  circle A14 centre (44.5, 8.5) radius 1.5
  circle A15 centre (12.7143, 13.5) radius 1.5
  circle A16 centre (6.3571, 13.5) radius 1.5
  circle A17 centre (38.1429, 13.5) radius 1.5
  circle A18 centre (25.4286, 13.5) radius 1.5
  circle A19 centre (44.5, 13.5) radius 1.5
  circle A20 centre (0, 13.5) radius 1.5
  circle A21 centre (19.0714, 13.5) radius 1.5
  circle A22 centre (31.7857, 13.5) radius 1.5
  circle A23 centre (12.7143, 18.5) radius 1.5
  circle A24 centre (6.3571, 18.5) radius 1.5
  circle A25 centre (38.1429, 18.5) radius 1.5
  circle A26 centre (25.4286, 18.5) radius 1.5
  circle A27 centre (44.5, 18.5) radius 1.5
  circle A28 centre (0, 18.5) radius 1.5
  circle A29 centre (19.0714, 18.5) radius 1.5
  circle A30 centre (31.7857, 18.5) radius 1.5
  point P0 (-44.5, 8.5)
  dimension "d27" = 7
  dimension "d29" = 40
  dimension "d38" = 1
  dimension "d74" = 3
  dimension "d77" = 89
  dimension "d78" = 5
  dimension "d79" = 7.5
  dimension "d80" = 7.5
  dimension "d102" = 0
  dimension "d103" = 10
  constraint horizontal L10
  constraint vertical L11
  constraint horizontal L12
  constraint vertical L13
  constraint midpoint L4 L14.end
  constraint perpendicular L6 L14
  constraint midpoint L14 P0
  constraint coincident P0 A0.centre
  measures "d27" distance of L6 L12
  measures "d29" distance of L10.start L10.end
  measures "d38" distance of L2 L10
  measures "d74" diameter of A0
  measures "d79" horizontal distance of L6.end P0
  measures "d80" horizontal distance of L6.start A14.centre
extrude "Extrude4" cut sketch "Sketch4" against normal up to surface (8 mm away) contours L2 L10 L11 L13 | L2 L11 L12 L13 | A0 | A1 | A2 | A3 | A4 | A5 | A6 | A7 | A8 | A9 | A10 | A11 | A12 | A13 | A14 | A15 | A16 | A17 | A18 | A19 | A20 | A21 | A22 | A23 | A24 | A25 | A26 | A27 | A28 | A29 | A30 bodies 1
sketch "Sketch5" plane through (60, 0, 0) normal (1, 0, 0) x (0, 0, -1)
  line L0 (-42, 0) -> (42, 0)
  line L1 (42, 0) -> (42, 31)
  line L2 (42, 31) -> (-42, 31)
  line L3 (-42, 31) -> (-42, 0)
  line L4 (19.45, 5) -> (25.55, 5)
  line L5 (19.45, 5) -> (25.55, 5)
  line L6 (-34, 5) -> (34, 5)
  line L7 (34, 5) -> (-34, 5)
  line L8 (-29.55, 5) -> (-23.45, 5)
  line L9 (-29.55, 5) -> (-23.45, 5)
  line L10 (-34, 31) -> (34, 31)
  line L11 (34, 31) -> (34, 13)
  line L12 (34, 13) -> (-34, 13)
  line L13 (-34, 13) -> (-34, 31)
  point P0 (-34, 31)
  point P1 (34, 31)
  dimension "d34" = 8
  constraint horizontal L10
  constraint vertical L11
  constraint horizontal L12
  constraint vertical L13
  constraint coincident L2 P0
  constraint coincident L13 P0
  constraint coincident L11 P1
  measures "d34" distance of L7 L12
extrude "Extrude5" cut sketch "Sketch5" against normal up to surface (8 mm away) contours L2 L10 L11 L12 L13 bodies 1
sketch "Sketch6" plane through (0, 31, 0) normal (0, 1, 0) x (-1, 0, 0)
  line L0 (-60, -34) -> (-60, -42)
  line L1 (-60, -42) -> (60, -42)
  line L2 (60, -42) -> (60, 42)
  line L3 (60, 42) -> (44.5, 42)
  line L4 (44.5, 42) -> (44.5, 34)
  line L5 (44.5, 34) -> (52, 34)
  line L6 (52, 34) -> (52, -34)
  line L7 (52, -34) -> (-60, -34)
  line L8 (-60, -34) -> (-60, -42) construction
  line L9 (-60, -34) -> (-60, -32) construction
  line L10 (-60, 34) -> (4.5, 34) construction
  line L11 (4.5, 34) -> (4.5, 42) construction
  line L12 (4.5, 42) -> (-60, 42) construction
  line L13 (-60, 42) -> (-60, 34) construction
  circle A0 centre (56, -38) radius 1.9
  circle A1 centre (-56, -38) radius 1.9
  circle A2 centre (-56, 38) radius 1.9
  circle A3 centre (56, 38) radius 1.9
  line L14 (-56, 38) -> (56, 38) construction
  line L15 (56, 38) -> (56, -38) construction
  line L16 (56, -38) -> (-56, -38) construction
  line L17 (-56, -38) -> (-56, 38) construction
  line L18 (-52, -34) -> (-52, 34) construction
  line L19 (-52, 34) -> (-60, 34) construction
  line L20 (-60, 34) -> (-60, -34) construction
  line L21 (-60, -34) -> (-52, -34) construction
  line L22 (52, -34) -> (60, -34) construction
  line L23 (52, -34) -> (52, -42) construction
  point P0 (-56, -34)
  point P1 (4.5, 38)
  point P2 (56, -34)
  point P3 (52, -38)
  dimension "d39" = 3.8
  dimension "d40" = 3.8
  dimension "d41" = 3.8
  dimension "d42" = 3.8
  constraint coincident L0.start L7.end
  constraint coincident L1 L0.end
  constraint perpendicular L1 L8
  constraint coincident L0 L9.end
  constraint coincident A2.centre L14.start
  constraint coincident A3.centre L14.end
  constraint parallel L3 L14
  constraint coincident A0.centre L15.end
  constraint coincident A1.centre L16.end
  constraint perpendicular L15 L16
  constraint perpendicular L14 L17
  constraint perpendicular L14 L15
  constraint midpoint L21 P0
  constraint coincident L17 P0
  constraint midpoint L11 P1
  constraint coincident L14 P1
  constraint coincident L6.end L7.start
  constraint coincident L2 L22.end
  constraint perpendicular L2 L22
  constraint coincident L1 L23.end
  constraint perpendicular L1 L23
  constraint midpoint L22 P2
  constraint midpoint L23 P3
  constraint coincident L16 P3
  constraint coincident L15 P2
  measures "d39" diameter of A0
  measures "d40" diameter of A1
  measures "d41" diameter of A2
  measures "d42" diameter of A3
extrude "Extrude6" cut sketch "Sketch6" against normal blind 10 contours A0 | A1 | A2 | A3 bodies 1
sketch "Sketch7" plane through (-60, 0, 0) normal (-1, 0, 0) x (0, 0, 1)
  line L0 (-42, 0) -> (42, 0)
  line L1 (42, 0) -> (42, 31)
  line L2 (42, 31) -> (-42, 31)
  line L3 (-42, 31) -> (-42, 0)
  line L4 (-19.45, 13) -> (-25.55, 13)
  line L5 (29.55, 13) -> (23.45, 13)
  line L6 (-25.55, 13) -> (29.55, 13) construction
  line L7 (-25.55, 5) -> (-19.45, 5)
  line L8 (-25.55, 5) -> (-19.45, 5)
  line L9 (34, 5) -> (-34, 5)
  line L10 (-34, 5) -> (34, 5)
  line L11 (23.45, 5) -> (29.55, 5)
  line L12 (23.45, 5) -> (29.55, 5)
  line L13 (-6, 16) -> (10, 16)
  line L14 (10, 16) -> (10, 5)
  line L15 (10, 5) -> (-6, 5)
  line L16 (-6, 5) -> (-6, 16)
  line L17 (2, 16) -> (2, 13) construction
  line L18 (-23.55, 13) -> (-21.45, 13)
  line L19 (25.45, 13) -> (27.55, 13)
  point P0 (2, 13)
  point P1 (2, 16)
  point P2 (0, 5)
  dimension "d54" = 16
  dimension "d55" = 3
  constraint coincident L4.end L6.start
  constraint coincident L5.start L6.end
  constraint midpoint L6 P0
  constraint horizontal L13
  constraint vertical L14
  constraint horizontal L15
  constraint vertical L16
  constraint midpoint L13 P1
  constraint coincident P1 L17.start
  constraint coincident P0 L17.end
  constraint vertical L17
  constraint midpoint L10 P2
  constraint coincident L15 P2
  measures "d54" distance of L13.start L13.end
  measures "d55" distance of P1 P0
extrude "Extrude7" cut sketch "Sketch7" against normal up to surface (8 mm away) contours L9 L10 L13 L14 L15 L16 bodies 1
sketch "Sketch8" plane through (0, 0, 0) normal (0, -1, 0) x (1, 0, 0)
  line L0 (-60, -42) -> (60, -42)
  line L1 (60, -42) -> (60, 42)
  line L2 (60, 42) -> (-60, 42)
  line L3 (-60, 42) -> (-60, -42)
  line L4 (-71.4, 47.15) -> (71.4, 47.15)
  line L5 (71.4, 47.15) -> (71.4, -47.15)
  line L6 (71.4, -47.15) -> (-71.4, -47.15)
  line L7 (-71.4, -47.15) -> (-71.4, 47.15)
  circle A0 centre (-66.9, -43.15) radius 2.25
  circle A1 centre (66.9, -43.15) radius 2.25
  circle A2 centre (66.9, 43.15) radius 2.25
  circle A3 centre (-66.9, 43.15) radius 2.25
  line L8 (-66.9, -43.15) -> (66.9, -43.15) construction
  line L9 (66.9, -43.15) -> (66.9, 43.15) construction
  line L10 (66.9, 43.15) -> (-66.9, 43.15) construction
  line L11 (-66.9, 43.15) -> (-66.9, -43.15) construction
  dimension "d60" = 142.8
  dimension "d61" = 94.3
  dimension "d62" = 71.4
  dimension "d63" = 47.15
  dimension "d64" = 4.5
  dimension "d65" = 4
  dimension "d66" = 4.5
  dimension "d67" = 4.5
  dimension "d68" = 4.5
  dimension "d69" = 4.5
  dimension "d70" = 4.5
  dimension "d71" = 4
  constraint horizontal L4
  constraint vertical L5
  constraint horizontal L6
  constraint vertical L7
  constraint coincident A0.centre L8.start
  constraint coincident A1.centre L8.end
  constraint coincident A2.centre L9.end
  constraint coincident A3.centre L10.end
  constraint horizontal L10
  constraint perpendicular L8 L11
  constraint perpendicular L8 L9
  constraint perpendicular L9 L10
  measures "d60" distance of L4.start L4.end
  measures "d61" distance of L4.start L6.end
  measures "d62" distance of origin L5
  measures "d63" distance of origin L4
  measures "d64" distance of L7 A0.centre
  measures "d65" distance of L6 A0.centre
  measures "d66" distance of L5 A1.centre
  measures "d67" diameter of A0
  measures "d68" diameter of A1
  measures "d69" diameter of A3
  measures "d70" diameter of A2
  measures "d71" distance of L4 A3.centre
extrude "Extrude8" add sketch "Sketch8" against normal blind 4 separate body makes body 2
sketch "Sketch10" plane through (0, 0, -42) normal (0, 0, -1) x (-1, 0, 0)
  line L0 (60, 31) -> (-60, 31)
  line L1 (-60, 0) -> (60, 0)
  circle A0 centre (-44.5, 8.5) radius 1.5
  circle A1 centre (-38.1429, 8.5) radius 1.5
  circle A2 centre (-31.7857, 8.5) radius 1.5
  circle A3 centre (-25.4286, 8.5) radius 1.5
  circle A4 centre (-19.0714, 8.5) radius 1.5
  circle A5 centre (-12.7143, 8.5) radius 1.5
  circle A6 centre (-6.3571, 8.5) radius 1.5
  circle A7 centre (0, 8.5) radius 1.5
  circle A8 centre (6.3571, 8.5) radius 1.5
  circle A9 centre (12.7143, 8.5) radius 1.5
  circle A10 centre (19.0714, 8.5) radius 1.5
  circle A11 centre (25.4286, 8.5) radius 1.5
  circle A12 centre (31.7857, 8.5) radius 1.5
  circle A13 centre (38.1429, 8.5) radius 1.5
  circle A14 centre (44.5, 8.5) radius 1.5
  circle A15 centre (25.4286, 13.5) radius 1.5
  circle A16 centre (6.3571, 13.5) radius 1.5
  circle A17 centre (44.5, 13.5) radius 1.5
  circle A18 centre (31.7857, 13.5) radius 1.5
  circle A19 centre (-31.7857, 13.5) radius 1.5
  circle A20 centre (19.0714, 13.5) radius 1.5
  circle A21 centre (38.1429, 13.5) radius 1.5
  circle A22 centre (0, 13.5) radius 1.5
  circle A23 centre (-19.0714, 13.5) radius 1.5
  circle A24 centre (12.7143, 13.5) radius 1.5
  circle A25 centre (-25.4286, 13.5) radius 1.5
  circle A26 centre (-12.7143, 13.5) radius 1.5
  circle A27 centre (-6.3571, 13.5) radius 1.5
  circle A28 centre (-38.1429, 13.5) radius 1.5
  circle A29 centre (-44.5, 13.5) radius 1.5
  circle A30 centre (25.4286, 18.5) radius 1.5
  circle A31 centre (6.3571, 18.5) radius 1.5
  circle A32 centre (44.5, 18.5) radius 1.5
  circle A33 centre (31.7857, 18.5) radius 1.5
  circle A34 centre (-31.7857, 18.5) radius 1.5
  circle A35 centre (19.0714, 18.5) radius 1.5
  circle A36 centre (38.1429, 18.5) radius 1.5
  circle A37 centre (0, 18.5) radius 1.5
  circle A38 centre (-19.0714, 18.5) radius 1.5
  circle A39 centre (12.7143, 18.5) radius 1.5
  circle A40 centre (-25.4286, 18.5) radius 1.5
  circle A41 centre (-12.7143, 18.5) radius 1.5
  circle A42 centre (-6.3571, 18.5) radius 1.5
  circle A43 centre (-38.1429, 18.5) radius 1.5
  circle A44 centre (-44.5, 18.5) radius 1.5
  line L2 (60, 0) -> (60, 31)
  line L3 (-60, 31) -> (-60, 0)
  dimension "d98" = 0
  dimension "d99" = 10
extrude "Extrude9" cut sketch "Sketch10" against normal up to surface (8 mm away) contours A0 | A1 | A2 | A3 | A4 | A5 | A6 | A7 | A8 | A9 | A10 | A11 | A12 | A13 | A14 | A15 | A16 | A17 | A18 | A19 | A20 | A21 | A22 | A23 | A24 | A25 | A26 | A27 | A28 | A29 | A30 | A31 | A32 | A33 | A34 | A35 | A36 | A37 | A38 | A39 | A40 | A41 | A42 | A43 | A44 bodies 1